Autodesk Fusion 360 part; units mm, degrees
(part 2 of 9)
  line L444 (-11.7276, 122.2942) -> (-7.3975, 119.7942)
  line L445 (-7.3975, 119.7942) -> (-3.0673, 122.2942)
  line L446 (-3.0673, 122.2942) -> (-3.0673, 127.2942)
  line L447 (-3.0673, 127.2942) -> (-7.3975, 129.7942)
  line L448 (-103.9199, 138.5933) -> (-108.25, 136.0933)
  line L449 (-108.25, 136.0933) -> (-108.25, 131.0933)
  line L450 (-108.25, 131.0933) -> (-103.9199, 128.5933)
  line L451 (-103.9199, 128.5933) -> (-99.5897, 131.0933)
  line L452 (-99.5897, 131.0933) -> (-99.5897, 136.0933)
  line L453 (-99.5897, 136.0933) -> (-103.9199, 138.5933)
  line L454 (-93.7596, 138.5933) -> (-98.0897, 136.0933)
  line L455 (-98.0897, 136.0933) -> (-98.0897, 131.0933)
  line L456 (-98.0897, 131.0933) -> (-93.7596, 128.5933)
  line L457 (-93.7596, 128.5933) -> (-89.4295, 131.0933)
  line L458 (-89.4295, 131.0933) -> (-89.4295, 136.0933)
  line L459 (-89.4295, 136.0933) -> (-93.7596, 138.5933)
  line L460 (-83.5994, 138.5933) -> (-87.9295, 136.0933)
  line L461 (-87.9295, 136.0933) -> (-87.9295, 131.0933)
  line L462 (-87.9295, 131.0933) -> (-83.5994, 128.5933)
  line L463 (-83.5994, 128.5933) -> (-79.2692, 131.0933)
  line L464 (-79.2692, 131.0933) -> (-79.2692, 136.0933)
  line L465 (-79.2692, 136.0933) -> (-83.5994, 138.5933)
  line L466 (-73.4391, 138.5933) -> (-77.7692, 136.0933)
  line L467 (-77.7692, 136.0933) -> (-77.7692, 131.0933)
  line L468 (-77.7692, 131.0933) -> (-73.4391, 128.5933)
  line L469 (-73.4391, 128.5933) -> (-69.109, 131.0933)
  line L470 (-69.109, 131.0933) -> (-69.109, 136.0933)
  line L471 (-69.109, 136.0933) -> (-73.4391, 138.5933)
  line L472 (-63.2789, 138.5933) -> (-67.609, 136.0933)
  line L473 (-67.609, 136.0933) -> (-67.609, 131.0933)
  line L474 (-67.609, 131.0933) -> (-63.2789, 128.5933)
  line L475 (-63.2789, 128.5933) -> (-58.9487, 131.0933)
  line L476 (-58.9487, 131.0933) -> (-58.9487, 136.0933)
  line L477 (-58.9487, 136.0933) -> (-63.2789, 138.5933)
  line L478 (-53.1186, 138.5933) -> (-57.4487, 136.0933)
  line L479 (-57.4487, 136.0933) -> (-57.4487, 131.0933)
  line L480 (-57.4487, 131.0933) -> (-53.1186, 128.5933)
  line L481 (-53.1186, 128.5933) -> (-48.7885, 131.0933)
  line L482 (-48.7885, 131.0933) -> (-48.7885, 136.0933)
  line L483 (-48.7885, 136.0933) -> (-53.1186, 138.5933)
  line L484 (-42.9584, 138.5933) -> (-47.2885, 136.0933)
  line L485 (-47.2885, 136.0933) -> (-47.2885, 131.0933)
  line L486 (-47.2885, 131.0933) -> (-42.9584, 128.5933)
  line L487 (-42.9584, 128.5933) -> (-38.6282, 131.0933)
  line L488 (-38.6282, 131.0933) -> (-38.6282, 136.0933)
  line L489 (-38.6282, 136.0933) -> (-42.9584, 138.5933)
  line L490 (-32.7981, 138.5933) -> (-37.1282, 136.0933)
  line L491 (-37.1282, 136.0933) -> (-37.1282, 131.0933)
  line L492 (-37.1282, 131.0933) -> (-32.7981, 128.5933)
  line L493 (-32.7981, 128.5933) -> (-28.468, 131.0933)
  line L494 (-28.468, 131.0933) -> (-28.468, 136.0933)
  line L495 (-28.468, 136.0933) -> (-32.7981, 138.5933)
  line L496 (-22.6378, 138.5933) -> (-26.968, 136.0933)
  line L497 (-26.968, 136.0933) -> (-26.968, 131.0933)
  line L498 (-26.968, 131.0933) -> (-22.6378, 128.5933)
  line L499 (-22.6378, 128.5933) -> (-18.3077, 131.0933)
  line L500 (-18.3077, 131.0933) -> (-18.3077, 136.0933)
  line L501 (-18.3077, 136.0933) -> (-22.6378, 138.5933)
  line L502 (-12.4776, 138.5933) -> (-16.8077, 136.0933)
  line L503 (-16.8077, 136.0933) -> (-16.8077, 131.0933)
  line L504 (-16.8077, 131.0933) -> (-12.4776, 128.5933)
  line L505 (-12.4776, 128.5933) -> (-8.1475, 131.0933)
  line L506 (-8.1475, 131.0933) -> (-8.1475, 136.0933)
  line L507 (-8.1475, 136.0933) -> (-12.4776, 138.5933)
  line L508 (-109, 147.3923) -> (-113.3301, 144.8923)
  line L509 (-113.3301, 144.8923) -> (-113.3301, 139.8923)
  line L510 (-113.3301, 139.8923) -> (-109, 137.3923)
  line L511 (-109, 137.3923) -> (-104.6699, 139.8923)
  line L512 (-104.6699, 139.8923) -> (-104.6699, 144.8923)
  line L513 (-104.6699, 144.8923) -> (-109, 147.3923)
  line L514 (-98.8397, 147.3923) -> (-103.1699, 144.8923)
  line L515 (-103.1699, 144.8923) -> (-103.1699, 139.8923)
  line L516 (-103.1699, 139.8923) -> (-98.8397, 137.3923)
  line L517 (-98.8397, 137.3923) -> (-94.5096, 139.8923)
  line L518 (-94.5096, 139.8923) -> (-94.5096, 144.8923)
  line L519 (-94.5096, 144.8923) -> (-98.8397, 147.3923)
  line L520 (-88.6795, 147.3923) -> (-93.0096, 144.8923)
  line L521 (-93.0096, 144.8923) -> (-93.0096, 139.8923)
  line L522 (-93.0096, 139.8923) -> (-88.6795, 137.3923)
  line L523 (-88.6795, 137.3923) -> (-84.3494, 139.8923)
  line L524 (-84.3494, 139.8923) -> (-84.3494, 144.8923)
  line L525 (-84.3494, 144.8923) -> (-88.6795, 147.3923)
  line L526 (-78.5192, 147.3923) -> (-82.8494, 144.8923)
  line L527 (-82.8494, 144.8923) -> (-82.8494, 139.8923)
  line L528 (-82.8494, 139.8923) -> (-78.5192, 137.3923)
  line L529 (-78.5192, 137.3923) -> (-74.1891, 139.8923)
  line L530 (-74.1891, 139.8923) -> (-74.1891, 144.8923)
  line L531 (-74.1891, 144.8923) -> (-78.5192, 147.3923)
  line L532 (-68.359, 147.3923) -> (-72.6891, 144.8923)
  line L533 (-72.6891, 144.8923) -> (-72.6891, 139.8923)
  line L534 (-72.6891, 139.8923) -> (-68.359, 137.3923)
  line L535 (-68.359, 137.3923) -> (-64.0289, 139.8923)
  line L536 (-64.0289, 139.8923) -> (-64.0289, 144.8923)
  line L537 (-64.0289, 144.8923) -> (-68.359, 147.3923)
  line L538 (-58.1987, 147.3923) -> (-62.5289, 144.8923)
  line L539 (-62.5289, 144.8923) -> (-62.5289, 139.8923)
  line L540 (-62.5289, 139.8923) -> (-58.1987, 137.3923)
  line L541 (-58.1987, 137.3923) -> (-53.8686, 139.8923)
  line L542 (-53.8686, 139.8923) -> (-53.8686, 144.8923)
  line L543 (-53.8686, 144.8923) -> (-58.1987, 147.3923)
  line L544 (-48.0385, 147.3923) -> (-52.3686, 144.8923)
  line L545 (-52.3686, 144.8923) -> (-52.3686, 139.8923)
  line L546 (-52.3686, 139.8923) -> (-48.0385, 137.3923)
  line L547 (-48.0385, 137.3923) -> (-43.7084, 139.8923)
  line L548 (-43.7084, 139.8923) -> (-43.7084, 144.8923)
  line L549 (-43.7084, 144.8923) -> (-48.0385, 147.3923)
  line L550 (-37.8782, 147.3923) -> (-42.2084, 144.8923)
  line L551 (-42.2084, 144.8923) -> (-42.2084, 139.8923)
  line L552 (-42.2084, 139.8923) -> (-37.8782, 137.3923)
  line L553 (-37.8782, 137.3923) -> (-33.5481, 139.8923)
  line L554 (-33.5481, 139.8923) -> (-33.5481, 144.8923)
  line L555 (-33.5481, 144.8923) -> (-37.8782, 147.3923)
  line L556 (-27.718, 147.3923) -> (-32.0481, 144.8923)
  line L557 (-32.0481, 144.8923) -> (-32.0481, 139.8923)
  line L558 (-32.0481, 139.8923) -> (-27.718, 137.3923)
  line L559 (-27.718, 137.3923) -> (-23.3878, 139.8923)
  line L560 (-23.3878, 139.8923) -> (-23.3878, 144.8923)
  line L561 (-23.3878, 144.8923) -> (-27.718, 147.3923)
  line L562 (-17.5577, 147.3923) -> (-21.8878, 144.8923)
  line L563 (-21.8878, 144.8923) -> (-21.8878, 139.8923)
  line L564 (-21.8878, 139.8923) -> (-17.5577, 137.3923)
  line L565 (-17.5577, 137.3923) -> (-13.2276, 139.8923)
  line L566 (-13.2276, 139.8923) -> (-13.2276, 144.8923)
  line L567 (-13.2276, 144.8923) -> (-17.5577, 147.3923)
  line L568 (-7.3975, 147.3923) -> (-11.7276, 144.8923)
  line L569 (-11.7276, 144.8923) -> (-11.7276, 139.8923)
  line L570 (-11.7276, 139.8923) -> (-7.3975, 137.3923)
  line L571 (-7.3975, 137.3923) -> (-3.0673, 139.8923)
  line L572 (-3.0673, 139.8923) -> (-3.0673, 144.8923)
  line L573 (-3.0673, 144.8923) -> (-7.3975, 147.3923)
  line L574 (-103.9199, 156.1913) -> (-108.25, 153.6913)
  line L575 (-108.25, 153.6913) -> (-108.25, 148.6913)
  line L576 (-108.25, 148.6913) -> (-103.9199, 146.1913)
  line L577 (-103.9199, 146.1913) -> (-99.5897, 148.6913)
  line L578 (-99.5897, 148.6913) -> (-99.5897, 153.6913)
  line L579 (-99.5897, 153.6913) -> (-103.9199, 156.1913)
  line L580 (-93.7596, 156.1913) -> (-98.0897, 153.6913)
  line L581 (-98.0897, 153.6913) -> (-98.0897, 148.6913)
  line L582 (-98.0897, 148.6913) -> (-93.7596, 146.1913)
  line L583 (-93.7596, 146.1913) -> (-89.4295, 148.6913)
  line L584 (-89.4295, 148.6913) -> (-89.4295, 153.6913)
  line L585 (-89.4295, 153.6913) -> (-93.7596, 156.1913)
  line L586 (-83.5994, 156.1913) -> (-87.9295, 153.6913)
  line L587 (-87.9295, 153.6913) -> (-87.9295, 148.6913)
  line L588 (-87.9295, 148.6913) -> (-83.5994, 146.1913)
  line L589 (-83.5994, 146.1913) -> (-79.2692, 148.6913)
  line L590 (-79.2692, 148.6913) -> (-79.2692, 153.6913)
  line L591 (-79.2692, 153.6913) -> (-83.5994, 156.1913)
  line L592 (-73.4391, 156.1913) -> (-77.7692, 153.6913)
  line L593 (-77.7692, 153.6913) -> (-77.7692, 148.6913)
  line L594 (-77.7692, 148.6913) -> (-73.4391, 146.1913)
  line L595 (-73.4391, 146.1913) -> (-69.109, 148.6913)
  line L596 (-69.109, 148.6913) -> (-69.109, 153.6913)
  line L597 (-69.109, 153.6913) -> (-73.4391, 156.1913)
  line L598 (-63.2789, 156.1913) -> (-67.609, 153.6913)
  line L599 (-67.609, 153.6913) -> (-67.609, 148.6913)
  line L600 (-67.609, 148.6913) -> (-63.2789, 146.1913)
  line L601 (-63.2789, 146.1913) -> (-58.9487, 148.6913)
  line L602 (-58.9487, 148.6913) -> (-58.9487, 153.6913)
  line L603 (-58.9487, 153.6913) -> (-63.2789, 156.1913)
  line L604 (-53.1186, 156.1913) -> (-57.4487, 153.6913)
  line L605 (-57.4487, 153.6913) -> (-57.4487, 148.6913)
  line L606 (-57.4487, 148.6913) -> (-53.1186, 146.1913)
  line L607 (-53.1186, 146.1913) -> (-48.7885, 148.6913)
  line L608 (-48.7885, 148.6913) -> (-48.7885, 153.6913)
  line L609 (-48.7885, 153.6913) -> (-53.1186, 156.1913)
  line L610 (-42.9584, 156.1913) -> (-47.2885, 153.6913)
  line L611 (-47.2885, 153.6913) -> (-47.2885, 148.6913)
  line L612 (-47.2885, 148.6913) -> (-42.9584, 146.1913)
  line L613 (-42.9584, 146.1913) -> (-38.6282, 148.6913)
  line L614 (-38.6282, 148.6913) -> (-38.6282, 153.6913)
  line L615 (-38.6282, 153.6913) -> (-42.9584, 156.1913)
  line L616 (-32.7981, 156.1913) -> (-37.1282, 153.6913)
  line L617 (-37.1282, 153.6913) -> (-37.1282, 148.6913)
  line L618 (-37.1282, 148.6913) -> (-32.7981, 146.1913)
  line L619 (-32.7981, 146.1913) -> (-28.468, 148.6913)
  line L620 (-28.468, 148.6913) -> (-28.468, 153.6913)
  line L621 (-28.468, 153.6913) -> (-32.7981, 156.1913)
  line L622 (-22.6378, 156.1913) -> (-26.968, 153.6913)
  line L623 (-26.968, 153.6913) -> (-26.968, 148.6913)
  line L624 (-26.968, 148.6913) -> (-22.6378, 146.1913)
  line L625 (-22.6378, 146.1913) -> (-18.3077, 148.6913)
  line L626 (-18.3077, 148.6913) -> (-18.3077, 153.6913)
  line L627 (-18.3077, 153.6913) -> (-22.6378, 156.1913)
  line L628 (-12.4776, 156.1913) -> (-16.8077, 153.6913)
  line L629 (-16.8077, 153.6913) -> (-16.8077, 148.6913)
  line L630 (-16.8077, 148.6913) -> (-12.4776, 146.1913)
  line L631 (-12.4776, 146.1913) -> (-8.1475, 148.6913)
  line L632 (-8.1475, 148.6913) -> (-8.1475, 153.6913)
  line L633 (-8.1475, 153.6913) -> (-12.4776, 156.1913)
extrude "拉伸21" cut sketch "草图20" against normal blind 3 contours L4 L5 L6 L7 L8 L9 | L10 L11 L12 L13 L14 L15 | L16 L17 L18 L19 L20 L21 | L22 L23 L24 L25 L26 L27 | L28 L29 L30 L31 L32 L33 | L34 L35 L36 L37 L38 L39 | L40 L41 L42 L43 L44 L45 | L46 L47 L48 L49 L50 L51 | L52 L53 L54 L55 L56 L57 | L58 L59 L60 L61 L62 L63 | L64 L65 L66 L67 L68 L69 | L70 L71 L72 L73 L74 L75 | L76 L77 L78 L79 L80 L81 | L82 L83 L84 L85 L86 L87 | L88 L89 L90 L91 L92 L93 | L94 L95 L96 L97 L98 L99 | L100 L101 L102 L103 L104 L105 | L106 L107 L108 L109 L110 L111 | L112 L113 L114 L115 L116 L117 | L118 L119 L120 L121 L122 L123 | L124 L125 L126 L127 L128 L129 | L130 L131 L132 L133 L134 L135 | L136 L137 L138 L139 L140 L141 | L142 L143 L144 L145 L146 L147 | L148 L149 L150 L151 L152 L153 | L154 L155 L156 L157 L158 L159 | L160 L161 L162 L163 L164 L165 | L166 L167 L168 L169 L170 L171 | L172 L173 L174 L175 L176 L177 | L178 L179 L180 L181 L182 L183 | L184 L185 L186 L187 L188 L189 | L190 L191 L192 L193 L194 L195 | L196 L197 L198 L199 L200 L201 | L202 L203 L204 L205 L206 L207 | L208 L209 L210 L211 L212 L213 | L214 L215 L216 L217 L218 L219 | L220 L221 L222 L223 L224 L225 | L226 L227 L228 L229 L230 L231 | L232 L233 L234 L235 L236 L237 | L238 L239 L240 L241 L242 L243 | L244 L245 L246 L247 L248 L249 | L250 L251 L252 L253 L254 L255 | L256 L257 L258 L259 L260 L261 | L262 L263 L264 L265 L266 L267 | L268 L269 L270 L271 L272 L273 | L274 L275 L276 L277 L278 L279 | L280 L281 L282 L283 L284 L285 | L286 L287 L288 L289 L290 L291 | L292 L293 L294 L295 L296 L297 | L298 L299 L300 L301 L302 L303 | L304 L305 L306 L307 L308 L309 | L310 L311 L312 L313 L314 L315 | L316 L317 L318 L319 L320 L321 | L322 L323 L324 L325 L326 L327 | L328 L329 L330 L331 L332 L333 | L334 L335 L336 L337 L338 L339 | L340 L341 L342 L343 L344 L345 | L346 L347 L348 L349 L350 L351 | L352 L353 L354 L355 L356 L357 | L358 L359 L360 L361 L362 L363 | L364 L365 L366 L367 L368 L369 | L370 L371 L372 L373 L374 L375 | L376 L377 L378 L379 L380 L381 | L382 L383 L384 L385 L386 L387 | L388 L389 L390 L391 L392 L393 | L394 L395 L396 L397 L398 L399 | L400 L401 L402 L403 L404 L405 | L406 L407 L408 L409 L410 L411 | L412 L413 L414 L415 L416 L417 | L418 L419 L420 L421 L422 L423 | L424 L425 L426 L427 L428 L429 | L430 L431 L432 L433 L434 L435 | L436 L437 L438 L439 L440 L441 | L442 L443 L444 L445 L446 L447 | L448 L449 L450 L451 L452 L453 | L454 L455 L456 L457 L458 L459 | L460 L461 L462 L463 L464 L465 | L466 L467 L468 L469 L470 L471 | L472 L473 L474 L475 L476 L477 | L478 L479 L480 L481 L482 L483 | L484 L485 L486 L487 L488 L489 | L490 L491 L492 L493 L494 L495 | L496 L497 L498 L499 L500 L501 | L502 L503 L504 L505 L506 L507 | L508 L509 L510 L511 L512 L513 | L514 L515 L516 L517 L518 L519 | L520 L521 L522 L523 L524 L525 | L526 L527 L528 L529 L530 L531 | L532 L533 L534 L535 L536 L537 | L538 L539 L540 L541 L542 L543 | L544 L545 L546 L547 L548 L549 | L550 L551 L552 L553 L554 L555 | L556 L557 L558 L559 L560 L561 | L562 L563 L564 L565 L566 L567 | L568 L569 L570 L571 L572 L573 | L574 L575 L576 L577 L578 L579 | L580 L581 L582 L583 L584 L585 | L586 L587 L588 L589 L590 L591 | L592 L593 L594 L595 L596 L597 | L598 L599 L600 L601 L602 L603 | L604 L605 L606 L607 L608 L609 | L610 L611 L612 L613 L614 L615 | L616 L617 L618 L619 L620 L621 | L622 L623 L624 L625 L626 L627 | L628 L629 L630 L631 L632 L633 bodies 1
sketch "草图21" plane through (0, 116, 0) normal (0, -1, 0) x (1, 0, 0)
  line L0 (3.9913, 65) -> (4, 65)
  line L1 (4, 65) -> (4, 160)
  line L2 (4, 160) -> (-116, 160)
  line L3 (-116, 160) -> (-116, 0)
  line L4 (-116, 0) -> (3.9913, 0)
  line L5 (3.9913, 0) -> (3.9913, 65)
  line L6 (-103.9199, 20.799) -> (-108.25, 18.299)
  line L7 (-108.25, 18.299) -> (-108.25, 13.299)
  line L8 (-108.25, 13.299) -> (-103.9199, 10.799)
  line L9 (-103.9199, 10.799) -> (-99.5897, 13.299)
  line L10 (-99.5897, 13.299) -> (-99.5897, 18.299)
  line L11 (-99.5897, 18.299) -> (-103.9199, 20.799)
  line L12 (-93.7596, 20.799) -> (-98.0897, 18.299)
  line L13 (-98.0897, 18.299) -> (-98.0897, 13.299)
  line L14 (-98.0897, 13.299) -> (-93.7596, 10.799)
  line L15 (-93.7596, 10.799) -> (-89.4295, 13.299)
  line L16 (-89.4295, 13.299) -> (-89.4295, 18.299)
  line L17 (-89.4295, 18.299) -> (-93.7596, 20.799)
  line L18 (-83.5994, 20.799) -> (-87.9295, 18.299)
  line L19 (-87.9295, 18.299) -> (-87.9295, 13.299)
  line L20 (-87.9295, 13.299) -> (-83.5994, 10.799)
  line L21 (-83.5994, 10.799) -> (-79.2692, 13.299)
  line L22 (-79.2692, 13.299) -> (-79.2692, 18.299)
  line L23 (-79.2692, 18.299) -> (-83.5994, 20.799)
  line L24 (-73.4391, 20.799) -> (-77.7692, 18.299)
  line L25 (-77.7692, 18.299) -> (-77.7692, 13.299)
  line L26 (-77.7692, 13.299) -> (-73.4391, 10.799)
  line L27 (-73.4391, 10.799) -> (-69.109, 13.299)
  line L28 (-69.109, 13.299) -> (-69.109, 18.299)
  line L29 (-69.109, 18.299) -> (-73.4391, 20.799)
  line L30 (-63.2789, 20.799) -> (-67.609, 18.299)
  line L31 (-67.609, 18.299) -> (-67.609, 13.299)
  line L32 (-67.609, 13.299) -> (-63.2789, 10.799)
  line L33 (-63.2789, 10.799) -> (-58.9487, 13.299)
  line L34 (-58.9487, 13.299) -> (-58.9487, 18.299)
  line L35 (-58.9487, 18.299) -> (-63.2789, 20.799)
  line L36 (-53.1186, 20.799) -> (-57.4487, 18.299)
  line L37 (-57.4487, 18.299) -> (-57.4487, 13.299)
  line L38 (-57.4487, 13.299) -> (-53.1186, 10.799)
  line L39 (-53.1186, 10.799) -> (-48.7885, 13.299)
  line L40 (-48.7885, 13.299) -> (-48.7885, 18.299)
  line L41 (-48.7885, 18.299) -> (-53.1186, 20.799)
  line L42 (-42.9584, 20.799) -> (-47.2885, 18.299)
  line L43 (-47.2885, 18.299) -> (-47.2885, 13.299)
  line L44 (-47.2885, 13.299) -> (-42.9584, 10.799)
  line L45 (-42.9584, 10.799) -> (-38.6282, 13.299)
  line L46 (-38.6282, 13.299) -> (-38.6282, 18.299)
  line L47 (-38.6282, 18.299) -> (-42.9584, 20.799)
  line L48 (-32.7981, 20.799) -> (-37.1282, 18.299)
  line L49 (-37.1282, 18.299) -> (-37.1282, 13.299)
  line L50 (-37.1282, 13.299) -> (-32.7981, 10.799)
  line L51 (-32.7981, 10.799) -> (-28.468, 13.299)
  line L52 (-28.468, 13.299) -> (-28.468, 18.299)
  line L53 (-28.468, 18.299) -> (-32.7981, 20.799)
  line L54 (-22.6378, 20.799) -> (-26.968, 18.299)
  line L55 (-26.968, 18.299) -> (-26.968, 13.299)
  line L56 (-26.968, 13.299) -> (-22.6378, 10.799)
  line L57 (-22.6378, 10.799) -> (-18.3077, 13.299)
  line L58 (-18.3077, 13.299) -> (-18.3077, 18.299)
  line L59 (-18.3077, 18.299) -> (-22.6378, 20.799)
  line L60 (-12.4776, 20.799) -> (-16.8077, 18.299)
  line L61 (-16.8077, 18.299) -> (-16.8077, 13.299)
  line L62 (-16.8077, 13.299) -> (-12.4776, 10.799)
  line L63 (-12.4776, 10.799) -> (-8.1475, 13.299)
  line L64 (-8.1475, 13.299) -> (-8.1475, 18.299)
  line L65 (-8.1475, 18.299) -> (-12.4776, 20.799)
  line L66 (-109, 29.5981) -> (-113.3301, 27.0981)
  line L67 (-113.3301, 27.0981) -> (-113.3301, 22.0981)
  line L68 (-113.3301, 22.0981) -> (-109, 19.5981)
  line L69 (-109, 19.5981) -> (-104.6699, 22.0981)
  line L70 (-104.6699, 22.0981) -> (-104.6699, 27.0981)
  line L71 (-104.6699, 27.0981) -> (-109, 29.5981)
  line L72 (-98.8397, 29.5981) -> (-103.1699, 27.0981)
  line L73 (-103.1699, 27.0981) -> (-103.1699, 22.0981)
  line L74 (-103.1699, 22.0981) -> (-98.8397, 19.5981)
  line L75 (-98.8397, 19.5981) -> (-94.5096, 22.0981)
  line L76 (-94.5096, 22.0981) -> (-94.5096, 27.0981)
  line L77 (-94.5096, 27.0981) -> (-98.8397, 29.5981)
  line L78 (-88.6795, 29.5981) -> (-93.0096, 27.0981)
  line L79 (-93.0096, 27.0981) -> (-93.0096, 22.0981)
  line L80 (-93.0096, 22.0981) -> (-88.6795, 19.5981)
  line L81 (-88.6795, 19.5981) -> (-84.3494, 22.0981)
  line L82 (-84.3494, 22.0981) -> (-84.3494, 27.0981)
  line L83 (-84.3494, 27.0981) -> (-88.6795, 29.5981)
  line L84 (-78.5192, 29.5981) -> (-82.8494, 27.0981)
  line L85 (-82.8494, 27.0981) -> (-82.8494, 22.0981)
  line L86 (-82.8494, 22.0981) -> (-78.5192, 19.5981)
  line L87 (-78.5192, 19.5981) -> (-74.1891, 22.0981)
  line L88 (-74.1891, 22.0981) -> (-74.1891, 27.0981)
  line L89 (-74.1891, 27.0981) -> (-78.5192, 29.5981)
  line L90 (-68.359, 29.5981) -> (-72.6891, 27.0981)
  line L91 (-72.6891, 27.0981) -> (-72.6891, 22.0981)
  line L92 (-72.6891, 22.0981) -> (-68.359, 19.5981)
  line L93 (-68.359, 19.5981) -> (-64.0289, 22.0981)
  line L94 (-64.0289, 22.0981) -> (-64.0289, 27.0981)
  line L95 (-64.0289, 27.0981) -> (-68.359, 29.5981)
  line L96 (-58.1987, 29.5981) -> (-62.5289, 27.0981)
  line L97 (-62.5289, 27.0981) -> (-62.5289, 22.0981)
  line L98 (-62.5289, 22.0981) -> (-58.1987, 19.5981)
  line L99 (-58.1987, 19.5981) -> (-53.8686, 22.0981)
  line L100 (-53.8686, 22.0981) -> (-53.8686, 27.0981)
  line L101 (-53.8686, 27.0981) -> (-58.1987, 29.5981)
  line L102 (-48.0385, 29.5981) -> (-52.3686, 27.0981)
  line L103 (-52.3686, 27.0981) -> (-52.3686, 22.0981)
  line L104 (-52.3686, 22.0981) -> (-48.0385, 19.5981)
  line L105 (-48.0385, 19.5981) -> (-43.7084, 22.0981)
  line L106 (-43.7084, 22.0981) -> (-43.7084, 27.0981)
  line L107 (-43.7084, 27.0981) -> (-48.0385, 29.5981)
  line L108 (-37.8782, 29.5981) -> (-42.2084, 27.0981)
  line L109 (-42.2084, 27.0981) -> (-42.2084, 22.0981)
  line L110 (-42.2084, 22.0981) -> (-37.8782, 19.5981)
  line L111 (-37.8782, 19.5981) -> (-33.5481, 22.0981)
  line L112 (-33.5481, 22.0981) -> (-33.5481, 27.0981)
  line L113 (-33.5481, 27.0981) -> (-37.8782, 29.5981)
  line L114 (-27.718, 29.5981) -> (-32.0481, 27.0981)
  line L115 (-32.0481, 27.0981) -> (-32.0481, 22.0981)
  line L116 (-32.0481, 22.0981) -> (-27.718, 19.5981)
  line L117 (-27.718, 19.5981) -> (-23.3878, 22.0981)
  line L118 (-23.3878, 22.0981) -> (-23.3878, 27.0981)
  line L119 (-23.3878, 27.0981) -> (-27.718, 29.5981)
  line L120 (-17.5577, 29.5981) -> (-21.8878, 27.0981)
  line L121 (-21.8878, 27.0981) -> (-21.8878, 22.0981)
  line L122 (-21.8878, 22.0981) -> (-17.5577, 19.5981)
  line L123 (-17.5577, 19.5981) -> (-13.2276, 22.0981)
  line L124 (-13.2276, 22.0981) -> (-13.2276, 27.0981)
  line L125 (-13.2276, 27.0981) -> (-17.5577, 29.5981)
  line L126 (-7.3975, 29.5981) -> (-11.7276, 27.0981)
  line L127 (-11.7276, 27.0981) -> (-11.7276, 22.0981)
  line L128 (-11.7276, 22.0981) -> (-7.3975, 19.5981)
  line L129 (-7.3975, 19.5981) -> (-3.0673, 22.0981)
  line L130 (-3.0673, 22.0981) -> (-3.0673, 27.0981)
  line L131 (-3.0673, 27.0981) -> (-7.3975, 29.5981)
  line L132 (-103.9199, 38.3971) -> (-108.25, 35.8971)
  line L133 (-108.25, 35.8971) -> (-108.25, 30.8971)
  line L134 (-108.25, 30.8971) -> (-103.9199, 28.3971)
  line L135 (-103.9199, 28.3971) -> (-99.5897, 30.8971)
  line L136 (-99.5897, 30.8971) -> (-99.5897, 35.8971)
  line L137 (-99.5897, 35.8971) -> (-103.9199, 38.3971)
  line L138 (-93.7596, 38.3971) -> (-98.0897, 35.8971)
  line L139 (-98.0897, 35.8971) -> (-98.0897, 30.8971)
  line L140 (-98.0897, 30.8971) -> (-93.7596, 28.3971)
  line L141 (-93.7596, 28.3971) -> (-89.4295, 30.8971)
  line L142 (-89.4295, 30.8971) -> (-89.4295, 35.8971)
  line L143 (-89.4295, 35.8971) -> (-93.7596, 38.3971)
  line L144 (-83.5994, 38.3971) -> (-87.9295, 35.8971)
  line L145 (-87.9295, 35.8971) -> (-87.9295, 30.8971)
  line L146 (-87.9295, 30.8971) -> (-83.5994, 28.3971)
  line L147 (-83.5994, 28.3971) -> (-79.2692, 30.8971)
  line L148 (-79.2692, 30.8971) -> (-79.2692, 35.8971)
  line L149 (-79.2692, 35.8971) -> (-83.5994, 38.3971)
  line L150 (-73.4391, 38.3971) -> (-77.7692, 35.8971)
  line L151 (-77.7692, 35.8971) -> (-77.7692, 30.8971)
  line L152 (-77.7692, 30.8971) -> (-73.4391, 28.3971)
  line L153 (-73.4391, 28.3971) -> (-69.109, 30.8971)
  line L154 (-69.109, 30.8971) -> (-69.109, 35.8971)
  line L155 (-69.109, 35.8971) -> (-73.4391, 38.3971)
  line L156 (-63.2789, 38.3971) -> (-67.609, 35.8971)
  line L157 (-67.609, 35.8971) -> (-67.609, 30.8971)
  line L158 (-67.609, 30.8971) -> (-63.2789, 28.3971)
  line L159 (-63.2789, 28.3971) -> (-58.9487, 30.8971)
  line L160 (-58.9487, 30.8971) -> (-58.9487, 35.8971)
  line L161 (-58.9487, 35.8971) -> (-63.2789, 38.3971)
  line L162 (-53.1186, 38.3971) -> (-57.4487, 35.8971)
  line L163 (-57.4487, 35.8971) -> (-57.4487, 30.8971)
  line L164 (-57.4487, 30.8971) -> (-53.1186, 28.3971)
  line L165 (-53.1186, 28.3971) -> (-48.7885, 30.8971)
  line L166 (-48.7885, 30.8971) -> (-48.7885, 35.8971)
  line L167 (-48.7885, 35.8971) -> (-53.1186, 38.3971)
  line L168 (-42.9584, 38.3971) -> (-47.2885, 35.8971)
  line L169 (-47.2885, 35.8971) -> (-47.2885, 30.8971)
  line L170 (-47.2885, 30.8971) -> (-42.9584, 28.3971)
  line L171 (-42.9584, 28.3971) -> (-38.6282, 30.8971)
  line L172 (-38.6282, 30.8971) -> (-38.6282, 35.8971)
  line L173 (-38.6282, 35.8971) -> (-42.9584, 38.3971)
  line L174 (-32.7981, 38.3971) -> (-37.1282, 35.8971)
  line L175 (-37.1282, 35.8971) -> (-37.1282, 30.8971)
  line L176 (-37.1282, 30.8971) -> (-32.7981, 28.3971)
  line L177 (-32.7981, 28.3971) -> (-28.468, 30.8971)
  line L178 (-28.468, 30.8971) -> (-28.468, 35.8971)
  line L179 (-28.468, 35.8971) -> (-32.7981, 38.3971)
  line L180 (-22.6378, 38.3971) -> (-26.968, 35.8971)
  line L181 (-26.968, 35.8971) -> (-26.968, 30.8971)
  line L182 (-26.968, 30.8971) -> (-22.6378, 28.3971)
  line L183 (-22.6378, 28.3971) -> (-18.3077, 30.8971)
  line L184 (-18.3077, 30.8971) -> (-18.3077, 35.8971)
  line L185 (-18.3077, 35.8971) -> (-22.6378, 38.3971)
  line L186 (-12.4776, 38.3971) -> (-16.8077, 35.8971)
  line L187 (-16.8077, 35.8971) -> (-16.8077, 30.8971)
  line L188 (-16.8077, 30.8971) -> (-12.4776, 28.3971)
  line L189 (-12.4776, 28.3971) -> (-8.1475, 30.8971)
  line L190 (-8.1475, 30.8971) -> (-8.1475, 35.8971)
  line L191 (-8.1475, 35.8971) -> (-12.4776, 38.3971)
  line L192 (-109, 47.1962) -> (-113.3301, 44.6962)
  line L193 (-113.3301, 44.6962) -> (-113.3301, 39.6962)
  line L194 (-113.3301, 39.6962) -> (-109, 37.1962)
  line L195 (-109, 37.1962) -> (-104.6699, 39.6962)
  line L196 (-104.6699, 39.6962) -> (-104.6699, 44.6962)
  line L197 (-104.6699, 44.6962) -> (-109, 47.1962)
  line L198 (-98.8397, 47.1962) -> (-103.1699, 44.6962)
  line L199 (-103.1699, 44.6962) -> (-103.1699, 39.6962)
  line L200 (-103.1699, 39.6962) -> (-98.8397, 37.1962)
  line L201 (-98.8397, 37.1962) -> (-94.5096, 39.6962)
  line L202 (-94.5096, 39.6962) -> (-94.5096, 44.6962)
  line L203 (-94.5096, 44.6962) -> (-98.8397, 47.1962)
  line L204 (-88.6795, 47.1962) -> (-93.0096, 44.6962)
  line L205 (-93.0096, 44.6962) -> (-93.0096, 39.6962)
  line L206 (-93.0096, 39.6962) -> (-88.6795, 37.1962)
  line L207 (-88.6795, 37.1962) -> (-84.3494, 39.6962)
  line L208 (-84.3494, 39.6962) -> (-84.3494, 44.6962)
  line L209 (-84.3494, 44.6962) -> (-88.6795, 47.1962)
  line L210 (-78.5192, 47.1962) -> (-82.8494, 44.6962)
  line L211 (-82.8494, 44.6962) -> (-82.8494, 39.6962)
  line L212 (-82.8494, 39.6962) -> (-78.5192, 37.1962)
  line L213 (-78.5192, 37.1962) -> (-74.1891, 39.6962)
  line L214 (-74.1891, 39.6962) -> (-74.1891, 44.6962)
  line L215 (-74.1891, 44.6962) -> (-78.5192, 47.1962)
  line L216 (-68.359, 47.1962) -> (-72.6891, 44.6962)
  line L217 (-72.6891, 44.6962) -> (-72.6891, 39.6962)
  line L218 (-72.6891, 39.6962) -> (-68.359, 37.1962)
  line L219 (-68.359, 37.1962) -> (-64.0289, 39.6962)
  line L220 (-64.0289, 39.6962) -> (-64.0289, 44.6962)
  line L221 (-64.0289, 44.6962) -> (-68.359, 47.1962)
  line L222 (-58.1987, 47.1962) -> (-62.5289, 44.6962)
  line L223 (-62.5289, 44.6962) -> (-62.5289, 39.6962)
  line L224 (-62.5289, 39.6962) -> (-58.1987, 37.1962)
  line L225 (-58.1987, 37.1962) -> (-53.8686, 39.6962)
  line L226 (-53.8686, 39.6962) -> (-53.8686, 44.6962)
  line L227 (-53.8686, 44.6962) -> (-58.1987, 47.1962)
  line L228 (-48.0385, 47.1962) -> (-52.3686, 44.6962)
  line L229 (-52.3686, 44.6962) -> (-52.3686, 39.6962)
  line L230 (-52.3686, 39.6962) -> (-48.0385, 37.1962)
  line L231 (-48.0385, 37.1962) -> (-43.7084, 39.6962)
  line L232 (-43.7084, 39.6962) -> (-43.7084, 44.6962)
  line L233 (-43.7084, 44.6962) -> (-48.0385, 47.1962)
  line L234 (-37.8782, 47.1962) -> (-42.2084, 44.6962)
  line L235 (-42.2084, 44.6962) -> (-42.2084, 39.6962)
  line L236 (-42.2084, 39.6962) -> (-37.8782, 37.1962)
  line L237 (-37.8782, 37.1962) -> (-33.5481, 39.6962)
  line L238 (-33.5481, 39.6962) -> (-33.5481, 44.6962)
  line L239 (-33.5481, 44.6962) -> (-37.8782, 47.1962)
  line L240 (-27.718, 47.1962) -> (-32.0481, 44.6962)
  line L241 (-32.0481, 44.6962) -> (-32.0481, 39.6962)
  line L242 (-32.0481, 39.6962) -> (-27.718, 37.1962)
  line L243 (-27.718, 37.1962) -> (-23.3878, 39.6962)
  line L244 (-23.3878, 39.6962) -> (-23.3878, 44.6962)
  line L245 (-23.3878, 44.6962) -> (-27.718, 47.1962)
  line L246 (-17.5577, 47.1962) -> (-21.8878, 44.6962)
  line L247 (-21.8878, 44.6962) -> (-21.8878, 39.6962)
  line L248 (-21.8878, 39.6962) -> (-17.5577, 37.1962)
  line L249 (-17.5577, 37.1962) -> (-13.2276, 39.6962)
  line L250 (-13.2276, 39.6962) -> (-13.2276, 44.6962)
  line L251 (-13.2276, 44.6962) -> (-17.5577, 47.1962)
  line L252 (-7.3975, 47.1962) -> (-11.7276, 44.6962)
  line L253 (-11.7276, 44.6962) -> (-11.7276, 39.6962)
  line L254 (-11.7276, 39.6962) -> (-7.3975, 37.1962)
  line L255 (-7.3975, 37.1962) -> (-3.0673, 39.6962)
  line L256 (-3.0673, 39.6962) -> (-3.0673, 44.6962)
  line L257 (-3.0673, 44.6962) -> (-7.3975, 47.1962)
  line L258 (-103.9199, 55.9952) -> (-108.25, 53.4952)
  line L259 (-108.25, 53.4952) -> (-108.25, 48.4952)
  line L260 (-108.25, 48.4952) -> (-103.9199, 45.9952)
  line L261 (-103.9199, 45.9952) -> (-99.5897, 48.4952)
  line L262 (-99.5897, 48.4952) -> (-99.5897, 53.4952)
  line L263 (-99.5897, 53.4952) -> (-103.9199, 55.9952)
  line L264 (-93.7596, 55.9952) -> (-98.0897, 53.4952)
  line L265 (-98.0897, 53.4952) -> (-98.0897, 48.4952)
  line L266 (-98.0897, 48.4952) -> (-93.7596, 45.9952)
  line L267 (-93.7596, 45.9952) -> (-89.4295, 48.4952)
  line L268 (-89.4295, 48.4952) -> (-89.4295, 53.4952)
  line L269 (-89.4295, 53.4952) -> (-93.7596, 55.9952)
  line L270 (-83.5994, 55.9952) -> (-87.9295, 53.4952)
  line L271 (-87.9295, 53.4952) -> (-87.9295, 48.4952)
  line L272 (-87.9295, 48.4952) -> (-83.5994, 45.9952)
  line L273 (-83.5994, 45.9952) -> (-79.2692, 48.4952)
  line L274 (-79.2692, 48.4952) -> (-79.2692, 53.4952)
  line L275 (-79.2692, 53.4952) -> (-83.5994, 55.9952)
  line L276 (-73.4391, 55.9952) -> (-77.7692, 53.4952)
  line L277 (-77.7692, 53.4952) -> (-77.7692, 48.4952)
  line L278 (-77.7692, 48.4952) -> (-73.4391, 45.9952)
  line L279 (-73.4391, 45.9952) -> (-69.109, 48.4952)
  line L280 (-69.109, 48.4952) -> (-69.109, 53.4952)
  line L281 (-69.109, 53.4952) -> (-73.4391, 55.9952)
  line L282 (-63.2789, 55.9952) -> (-67.609, 53.4952)
  line L283 (-67.609, 53.4952) -> (-67.609, 48.4952)
  line L284 (-67.609, 48.4952) -> (-63.2789, 45.9952)
  line L285 (-63.2789, 45.9952) -> (-58.9487, 48.4952)
  line L286 (-58.9487, 48.4952) -> (-58.9487, 53.4952)
  line L287 (-58.9487, 53.4952) -> (-63.2789, 55.9952)
  line L288 (-53.1186, 55.9952) -> (-57.4487, 53.4952)
  line L289 (-57.4487, 53.4952) -> (-57.4487, 48.4952)
  line L290 (-57.4487, 48.4952) -> (-53.1186, 45.9952)
  line L291 (-53.1186, 45.9952) -> (-48.7885, 48.4952)
  line L292 (-48.7885, 48.4952) -> (-48.7885, 53.4952)
  line L293 (-48.7885, 53.4952) -> (-53.1186, 55.9952)
  line L294 (-42.9584, 55.9952) -> (-47.2885, 53.4952)
  line L295 (-47.2885, 53.4952) -> (-47.2885, 48.4952)
  line L296 (-47.2885, 48.4952) -> (-42.9584, 45.9952)
  line L297 (-42.9584, 45.9952) -> (-38.6282, 48.4952)
  line L298 (-38.6282, 48.4952) -> (-38.6282, 53.4952)
  line L299 (-38.6282, 53.4952) -> (-42.9584, 55.9952)
  line L300 (-32.7981, 55.9952) -> (-37.1282, 53.4952)
  line L301 (-37.1282, 53.4952) -> (-37.1282, 48.4952)
  line L302 (-37.1282, 48.4952) -> (-32.7981, 45.9952)
  line L303 (-32.7981, 45.9952) -> (-28.468, 48.4952)
  line L304 (-28.468, 48.4952) -> (-28.468, 53.4952)
  line L305 (-28.468, 53.4952) -> (-32.7981, 55.9952)
  line L306 (-22.6378, 55.9952) -> (-26.968, 53.4952)
  line L307 (-26.968, 53.4952) -> (-26.968, 48.4952)
  line L308 (-26.968, 48.4952) -> (-22.6378, 45.9952)
  line L309 (-22.6378, 45.9952) -> (-18.3077, 48.4952)
  line L310 (-18.3077, 48.4952) -> (-18.3077, 53.4952)
  line L311 (-18.3077, 53.4952) -> (-22.6378, 55.9952)
  line L312 (-12.4776, 55.9952) -> (-16.8077, 53.4952)
  line L313 (-16.8077, 53.4952) -> (-16.8077, 48.4952)
  line L314 (-16.8077, 48.4952) -> (-12.4776, 45.9952)
  line L315 (-12.4776, 45.9952) -> (-8.1475, 48.4952)
  line L316 (-8.1475, 48.4952) -> (-8.1475, 53.4952)
  line L317 (-8.1475, 53.4952) -> (-12.4776, 55.9952)
  line L318 (-109, 64.7942) -> (-113.3301, 62.2942)
  line L319 (-113.3301, 62.2942) -> (-113.3301, 57.2942)
  line L320 (-113.3301, 57.2942) -> (-109, 54.7942)
  line L321 (-109, 54.7942) -> (-104.6699, 57.2942)
  line L322 (-104.6699, 57.2942) -> (-104.6699, 62.2942)
  line L323 (-104.6699, 62.2942) -> (-109, 64.7942)
  line L324 (-98.8397, 64.7942) -> (-103.1699, 62.2942)
  line L325 (-103.1699, 62.2942) -> (-103.1699, 57.2942)
  line L326 (-103.1699, 57.2942) -> (-98.8397, 54.7942)
  line L327 (-98.8397, 54.7942) -> (-94.5096, 57.2942)
  line L328 (-94.5096, 57.2942) -> (-94.5096, 62.2942)
  line L329 (-94.5096, 62.2942) -> (-98.8397, 64.7942)
  line L330 (-88.6795, 64.7942) -> (-93.0096, 62.2942)
  line L331 (-93.0096, 62.2942) -> (-93.0096, 57.2942)
  line L332 (-93.0096, 57.2942) -> (-88.6795, 54.7942)
  line L333 (-88.6795, 54.7942) -> (-84.3494, 57.2942)
  line L334 (-84.3494, 57.2942) -> (-84.3494, 62.2942)
  line L335 (-84.3494, 62.2942) -> (-88.6795, 64.7942)
  line L336 (-78.5192, 64.7942) -> (-82.8494, 62.2942)
  line L337 (-82.8494, 62.2942) -> (-82.8494, 57.2942)
  line L338 (-82.8494, 57.2942) -> (-78.5192, 54.7942)
  line L339 (-78.5192, 54.7942) -> (-74.1891, 57.2942)
  line L340 (-74.1891, 57.2942) -> (-74.1891, 62.2942)
  line L341 (-74.1891, 62.2942) -> (-78.5192, 64.7942)
  line L342 (-68.359, 64.7942) -> (-72.6891, 62.2942)
  line L343 (-72.6891, 62.2942) -> (-72.6891, 57.2942)
  line L344 (-72.6891, 57.2942) -> (-68.359, 54.7942)
  line L345 (-68.359, 54.7942) -> (-64.0289, 57.2942)
  line L346 (-64.0289, 57.2942) -> (-64.0289, 62.2942)
  line L347 (-64.0289, 62.2942) -> (-68.359, 64.7942)
  line L348 (-58.1987, 64.7942) -> (-62.5289, 62.2942)
  line L349 (-62.5289, 62.2942) -> (-62.5289, 57.2942)
  line L350 (-62.5289, 57.2942) -> (-58.1987, 54.7942)
  line L351 (-58.1987, 54.7942) -> (-53.8686, 57.2942)
  line L352 (-53.8686, 57.2942) -> (-53.8686, 62.2942)
  line L353 (-53.8686, 62.2942) -> (-58.1987, 64.7942)
  line L354 (-48.0385, 64.7942) -> (-52.3686, 62.2942)
  line L355 (-52.3686, 62.2942) -> (-52.3686, 57.2942)
  line L356 (-52.3686, 57.2942) -> (-48.0385, 54.7942)
  line L357 (-48.0385, 54.7942) -> (-43.7084, 57.2942)
  line L358 (-43.7084, 57.2942) -> (-43.7084, 62.2942)
  line L359 (-43.7084, 62.2942) -> (-48.0385, 64.7942)
  line L360 (-37.8782, 64.7942) -> (-42.2084, 62.2942)
  line L361 (-42.2084, 62.2942) -> (-42.2084, 57.2942)
  line L362 (-42.2084, 57.2942) -> (-37.8782, 54.7942)
  line L363 (-37.8782, 54.7942) -> (-33.5481, 57.2942)
  line L364 (-33.5481, 57.2942) -> (-33.5481, 62.2942)
  line L365 (-33.5481, 62.2942) -> (-37.8782, 64.7942)
  line L366 (-27.718, 64.7942) -> (-32.0481, 62.2942)
  line L367 (-32.0481, 62.2942) -> (-32.0481, 57.2942)
  line L368 (-32.0481, 57.2942) -> (-27.718, 54.7942)
  line L369 (-27.718, 54.7942) -> (-23.3878, 57.2942)
  line L370 (-23.3878, 57.2942) -> (-23.3878, 62.2942)
  line L371 (-23.3878, 62.2942) -> (-27.718, 64.7942)
  line L372 (-17.5577, 64.7942) -> (-21.8878, 62.2942)
  line L373 (-21.8878, 62.2942) -> (-21.8878, 57.2942)
  line L374 (-21.8878, 57.2942) -> (-17.5577, 54.7942)
  line L375 (-17.5577, 54.7942) -> (-13.2276, 57.2942)
  line L376 (-13.2276, 57.2942) -> (-13.2276, 62.2942)
  line L377 (-13.2276, 62.2942) -> (-17.5577, 64.7942)
  line L378 (-7.3975, 64.7942) -> (-11.7276, 62.2942)
  line L379 (-11.7276, 62.2942) -> (-11.7276, 57.2942)
  line L380 (-11.7276, 57.2942) -> (-7.3975, 54.7942)
  line L381 (-7.3975, 54.7942) -> (-3.0673, 57.2942)
  line L382 (-3.0673, 57.2942) -> (-3.0673, 62.2942)
  line L383 (-3.0673, 62.2942) -> (-7.3975, 64.7942)
  line L384 (-103.9199, 73.5933) -> (-108.25, 71.0933)
  line L385 (-108.25, 71.0933) -> (-108.25, 66.0933)
  line L386 (-108.25, 66.0933) -> (-103.9199, 63.5933)
  line L387 (-103.9199, 63.5933) -> (-99.5897, 66.0933)
  line L388 (-99.5897, 66.0933) -> (-99.5897, 71.0933)
  line L389 (-99.5897, 71.0933) -> (-103.9199, 73.5933)
  line L390 (-93.7596, 73.5933) -> (-98.0897, 71.0933)
  line L391 (-98.0897, 71.0933) -> (-98.0897, 66.0933)
  line L392 (-98.0897, 66.0933) -> (-93.7596, 63.5933)
  line L393 (-93.7596, 63.5933) -> (-89.4295, 66.0933)
  line L394 (-89.4295, 66.0933) -> (-89.4295, 71.0933)
  line L395 (-89.4295, 71.0933) -> (-93.7596, 73.5933)
  line L396 (-83.5994, 73.5933) -> (-87.9295, 71.0933)
  line L397 (-87.9295, 71.0933) -> (-87.9295, 66.0933)
  line L398 (-87.9295, 66.0933) -> (-83.5994, 63.5933)
  line L399 (-83.5994, 63.5933) -> (-79.2692, 66.0933)
  line L400 (-79.2692, 66.0933) -> (-79.2692, 71.0933)
  line L401 (-79.2692, 71.0933) -> (-83.5994, 73.5933)
  line L402 (-73.4391, 73.5933) -> (-77.7692, 71.0933)
  line L403 (-77.7692, 71.0933) -> (-77.7692, 66.0933)
  line L404 (-77.7692, 66.0933) -> (-73.4391, 63.5933)
  line L405 (-73.4391, 63.5933) -> (-69.109, 66.0933)
  line L406 (-69.109, 66.0933) -> (-69.109, 71.0933)
  line L407 (-69.109, 71.0933) -> (-73.4391, 73.5933)
  line L408 (-63.2789, 73.5933) -> (-67.609, 71.0933)
  line L409 (-67.609, 71.0933) -> (-67.609, 66.0933)
  line L410 (-67.609, 66.0933) -> (-63.2789, 63.5933)
  line L411 (-63.2789, 63.5933) -> (-58.9487, 66.0933)
  line L412 (-58.9487, 66.0933) -> (-58.9487, 71.0933)
  line L413 (-58.9487, 71.0933) -> (-63.2789, 73.5933)
  line L414 (-53.1186, 73.5933) -> (-57.4487, 71.0933)
  line L415 (-57.4487, 71.0933) -> (-57.4487, 66.0933)
  line L416 (-57.4487, 66.0933) -> (-53.1186, 63.5933)
  line L417 (-53.1186, 63.5933) -> (-48.7885, 66.0933)
  line L418 (-48.7885, 66.0933) -> (-48.7885, 71.0933)
  line L419 (-48.7885, 71.0933) -> (-53.1186, 73.5933)
  line L420 (-42.9584, 73.5933) -> (-47.2885, 71.0933)
  line L421 (-47.2885, 71.0933) -> (-47.2885, 66.0933)
  line L422 (-47.2885, 66.0933) -> (-42.9584, 63.5933)
  line L423 (-42.9584, 63.5933) -> (-38.6282, 66.0933)
  line L424 (-38.6282, 66.0933) -> (-38.6282, 71.0933)
  line L425 (-38.6282, 71.0933) -> (-42.9584, 73.5933)
  line L426 (-32.7981, 73.5933) -> (-37.1282, 71.0933)
  line L427 (-37.1282, 71.0933) -> (-37.1282, 66.0933)
  line L428 (-37.1282, 66.0933) -> (-32.7981, 63.5933)
  line L429 (-32.7981, 63.5933) -> (-28.468, 66.0933)
  line L430 (-28.468, 66.0933) -> (-28.468, 71.0933)
  line L431 (-28.468, 71.0933) -> (-32.7981, 73.5933)
  line L432 (-22.6378, 73.5933) -> (-26.968, 71.0933)
  line L433 (-26.968, 71.0933) -> (-26.968, 66.0933)
  line L434 (-26.968, 66.0933) -> (-22.6378, 63.5933)
  line L435 (-22.6378, 63.5933) -> (-18.3077, 66.0933)
  line L436 (-18.3077, 66.0933) -> (-18.3077, 71.0933)
  line L437 (-18.3077, 71.0933) -> (-22.6378, 73.5933)
  line L438 (-12.4776, 73.5933) -> (-16.8077, 71.0933)
  line L439 (-16.8077, 71.0933) -> (-16.8077, 66.0933)
  line L440 (-16.8077, 66.0933) -> (-12.4776, 63.5933)
  line L441 (-12.4776, 63.5933) -> (-8.1475, 66.0933)
  line L442 (-8.1475, 66.0933) -> (-8.1475, 71.0933)
  line L443 (-8.1475, 71.0933) -> (-12.4776, 73.5933)
  line L444 (-109, 82.3923) -> (-113.3301, 79.8923)
  line L445 (-113.3301, 79.8923) -> (-113.3301, 74.8923)
  line L446 (-113.3301, 74.8923) -> (-109, 72.3923)
  line L447 (-109, 72.3923) -> (-104.6699, 74.8923)
  line L448 (-104.6699, 74.8923) -> (-104.6699, 79.8923)
  line L449 (-104.6699, 79.8923) -> (-109, 82.3923)
  line L450 (-98.8397, 82.3923) -> (-103.1699, 79.8923)
  line L451 (-103.1699, 79.8923) -> (-103.1699, 74.8923)
  line L452 (-103.1699, 74.8923) -> (-98.8397, 72.3923)
  line L453 (-98.8397, 72.3923) -> (-94.5096, 74.8923)
  line L454 (-94.5096, 74.8923) -> (-94.5096, 79.8923)
  line L455 (-94.5096, 79.8923) -> (-98.8397, 82.3923)
  line L456 (-88.6795, 82.3923) -> (-93.0096, 79.8923)
  line L457 (-93.0096, 79.8923) -> (-93.0096, 74.8923)
  line L458 (-93.0096, 74.8923) -> (-88.6795, 72.3923)
  line L459 (-88.6795, 72.3923) -> (-84.3494, 74.8923)
  line L460 (-84.3494, 74.8923) -> (-84.3494, 79.8923)
  line L461 (-84.3494, 79.8923) -> (-88.6795, 82.3923)
  line L462 (-78.5192, 82.3923) -> (-82.8494, 79.8923)
  line L463 (-82.8494, 79.8923) -> (-82.8494, 74.8923)
  line L464 (-82.8494, 74.8923) -> (-78.5192, 72.3923)
  line L465 (-78.5192, 72.3923) -> (-74.1891, 74.8923)
  line L466 (-74.1891, 74.8923) -> (-74.1891, 79.8923)
  line L467 (-74.1891, 79.8923) -> (-78.5192, 82.3923)
  line L468 (-68.359, 82.3923) -> (-72.6891, 79.8923)
  line L469 (-72.6891, 79.8923) -> (-72.6891, 74.8923)
  line L470 (-72.6891, 74.8923) -> (-68.359, 72.3923)
  line L471 (-68.359, 72.3923) -> (-64.0289, 74.8923)
  line L472 (-64.0289, 74.8923) -> (-64.0289, 79.8923)
  line L473 (-64.0289, 79.8923) -> (-68.359, 82.3923)
  line L474 (-58.1987, 82.3923) -> (-62.5289, 79.8923)
  line L475 (-62.5289, 79.8923) -> (-62.5289, 74.8923)
  line L476 (-62.5289, 74.8923) -> (-58.1987, 72.3923)
  line L477 (-58.1987, 72.3923) -> (-53.8686, 74.8923)
  line L478 (-53.8686, 74.8923) -> (-53.8686, 79.8923)
  line L479 (-53.8686, 79.8923) -> (-58.1987, 82.3923)
  line L480 (-48.0385, 82.3923) -> (-52.3686, 79.8923)
  line L481 (-52.3686, 79.8923) -> (-52.3686, 74.8923)
  line L482 (-52.3686, 74.8923) -> (-48.0385, 72.3923)
  line L483 (-48.0385, 72.3923) -> (-43.7084, 74.8923)
  line L484 (-43.7084, 74.8923) -> (-43.7084, 79.8923)
  line L485 (-43.7084, 79.8923) -> (-48.0385, 82.3923)
  line L486 (-37.8782, 82.3923) -> (-42.2084, 79.8923)
  line L487 (-42.2084, 79.8923) -> (-42.2084, 74.8923)
  line L488 (-42.2084, 74.8923) -> (-37.8782, 72.3923)
  line L489 (-37.8782, 72.3923) -> (-33.5481, 74.8923)
  line L490 (-33.5481, 74.8923) -> (-33.5481, 79.8923)
  line L491 (-33.5481, 79.8923) -> (-37.8782, 82.3923)
  line L492 (-27.718, 82.3923) -> (-32.0481, 79.8923)
  line L493 (-32.0481, 79.8923) -> (-32.0481, 74.8923)
  line L494 (-32.0481, 74.8923) -> (-27.718, 72.3923)
  line L495 (-27.718, 72.3923) -> (-23.3878, 74.8923)
  line L496 (-23.3878, 74.8923) -> (-23.3878, 79.8923)
  line L497 (-23.3878, 79.8923) -> (-27.718, 82.3923)
  line L498 (-17.5577, 82.3923) -> (-21.8878, 79.8923)
  line L499 (-21.8878, 79.8923) -> (-21.8878, 74.8923)
  line L500 (-21.8878, 74.8923) -> (-17.5577, 72.3923)
  line L501 (-17.5577, 72.3923) -> (-13.2276, 74.8923)
  line L502 (-13.2276, 74.8923) -> (-13.2276, 79.8923)
  line L503 (-13.2276, 79.8923) -> (-17.5577, 82.3923)
  line L504 (-7.3975, 82.3923) -> (-11.7276, 79.8923)
  line L505 (-11.7276, 79.8923) -> (-11.7276, 74.8923)
  line L506 (-11.7276, 74.8923) -> (-7.3975, 72.3923)
  line L507 (-7.3975, 72.3923) -> (-3.0673, 74.8923)
  line L508 (-3.0673, 74.8923) -> (-3.0673, 79.8923)
  line L509 (-3.0673, 79.8923) -> (-7.3975, 82.3923)
  line L510 (-103.9199, 91.1913) -> (-108.25, 88.6913)
  line L511 (-108.25, 88.6913) -> (-108.25, 83.6913)
  line L512 (-108.25, 83.6913) -> (-103.9199, 81.1913)
  line L513 (-103.9199, 81.1913) -> (-99.5897, 83.6913)
  line L514 (-99.5897, 83.6913) -> (-99.5897, 88.6913)
  line L515 (-99.5897, 88.6913) -> (-103.9199, 91.1913)
  line L516 (-93.7596, 91.1913) -> (-98.0897, 88.6913)
  line L517 (-98.0897, 88.6913) -> (-98.0897, 83.6913)
  line L518 (-98.0897, 83.6913) -> (-93.7596, 81.1913)
  line L519 (-93.7596, 81.1913) -> (-89.4295, 83.6913)
  line L520 (-89.4295, 83.6913) -> (-89.4295, 88.6913)
  line L521 (-89.4295, 88.6913) -> (-93.7596, 91.1913)
  line L522 (-83.5994, 91.1913) -> (-87.9295, 88.6913)
  line L523 (-87.9295, 88.6913) -> (-87.9295, 83.6913)
  line L524 (-87.9295, 83.6913) -> (-83.5994, 81.1913)
  line L525 (-83.5994, 81.1913) -> (-79.2692, 83.6913)
  line L526 (-79.2692, 83.6913) -> (-79.2692, 88.6913)
  line L527 (-79.2692, 88.6913) -> (-83.5994, 91.1913)
  line L528 (-73.4391, 91.1913) -> (-77.7692, 88.6913)
  line L529 (-77.7692, 88.6913) -> (-77.7692, 83.6913)
  line L530 (-77.7692, 83.6913) -> (-73.4391, 81.1913)
  line L531 (-73.4391, 81.1913) -> (-69.109, 83.6913)
  line L532 (-69.109, 83.6913) -> (-69.109, 88.6913)
  line L533 (-69.109, 88.6913) -> (-73.4391, 91.1913)
  line L534 (-63.2789, 91.1913) -> (-67.609, 88.6913)
  line L535 (-67.609, 88.6913) -> (-67.609, 83.6913)
  line L536 (-67.609, 83.6913) -> (-63.2789, 81.1913)
  line L537 (-63.2789, 81.1913) -> (-58.9487, 83.6913)
  line L538 (-58.9487, 83.6913) -> (-58.9487, 88.6913)
  line L539 (-58.9487, 88.6913) -> (-63.2789, 91.1913)
  line L540 (-53.1186, 91.1913) -> (-57.4487, 88.6913)
  line L541 (-57.4487, 88.6913) -> (-57.4487, 83.6913)
  line L542 (-57.4487, 83.6913) -> (-53.1186, 81.1913)
  line L543 (-53.1186, 81.1913) -> (-48.7885, 83.6913)
  line L544 (-48.7885, 83.6913) -> (-48.7885, 88.6913)
  line L545 (-48.7885, 88.6913) -> (-53.1186, 91.1913)
  line L546 (-42.9584, 91.1913) -> (-47.2885, 88.6913)
  line L547 (-47.2885, 88.6913) -> (-47.2885, 83.6913)
  line L548 (-47.2885, 83.6913) -> (-42.9584, 81.1913)
  line L549 (-42.9584, 81.1913) -> (-38.6282, 83.6913)
  line L550 (-38.6282, 83.6913) -> (-38.6282, 88.6913)
  line L551 (-38.6282, 88.6913) -> (-42.9584, 91.1913)
  line L552 (-32.7981, 91.1913) -> (-37.1282, 88.6913)
  line L553 (-37.1282, 88.6913) -> (-37.1282, 83.6913)
  line L554 (-37.1282, 83.6913) -> (-32.7981, 81.1913)
  line L555 (-32.7981, 81.1913) -> (-28.468, 83.6913)
  line L556 (-28.468, 83.6913) -> (-28.468, 88.6913)
  line L557 (-28.468, 88.6913) -> (-32.7981, 91.1913)
  line L558 (-22.6378, 91.1913) -> (-26.968, 88.6913)
  line L559 (-26.968, 88.6913) -> (-26.968, 83.6913)
  line L560 (-26.968, 83.6913) -> (-22.6378, 81.1913)
  line L561 (-22.6378, 81.1913) -> (-18.3077, 83.6913)
  line L562 (-18.3077, 83.6913) -> (-18.3077, 88.6913)
  line L563 (-18.3077, 88.6913) -> (-22.6378, 91.1913)
  line L564 (-12.4776, 91.1913) -> (-16.8077, 88.6913)
  line L565 (-16.8077, 88.6913) -> (-16.8077, 83.6913)
  line L566 (-16.8077, 83.6913) -> (-12.4776, 81.1913)
  line L567 (-12.4776, 81.1913) -> (-8.1475, 83.6913)
  line L568 (-8.1475, 83.6913) -> (-8.1475, 88.6913)
  line L569 (-8.1475, 88.6913) -> (-12.4776, 91.1913)
  line L570 (-109, 99.9904) -> (-113.3301, 97.4904)
  line L571 (-113.3301, 97.4904) -> (-113.3301, 92.4904)
  line L572 (-113.3301, 92.4904) -> (-109, 89.9904)
  line L573 (-109, 89.9904) -> (-104.6699, 92.4904)
  line L574 (-104.6699, 92.4904) -> (-104.6699, 97.4904)
  line L575 (-104.6699, 97.4904) -> (-109, 99.9904)
  line L576 (-98.8397, 99.9904) -> (-103.1699, 97.4904)
  line L577 (-103.1699, 97.4904) -> (-103.1699, 92.4904)
  line L578 (-103.1699, 92.4904) -> (-98.8397, 89.9904)
  line L579 (-98.8397, 89.9904) -> (-94.5096, 92.4904)
  line L580 (-94.5096, 92.4904) -> (-94.5096, 97.4904)
  line L581 (-94.5096, 97.4904) -> (-98.8397, 99.9904)
  line L582 (-88.6795, 99.9904) -> (-93.0096, 97.4904)
  line L583 (-93.0096, 97.4904) -> (-93.0096, 92.4904)
  line L584 (-93.0096, 92.4904) -> (-88.6795, 89.9904)
  line L585 (-88.6795, 89.9904) -> (-84.3494, 92.4904)
  line L586 (-84.3494, 92.4904) -> (-84.3494, 97.4904)
  line L587 (-84.3494, 97.4904) -> (-88.6795, 99.9904)
  line L588 (-78.5192, 99.9904) -> (-82.8494, 97.4904)
  line L589 (-82.8494, 97.4904) -> (-82.8494, 92.4904)
  line L590 (-82.8494, 92.4904) -> (-78.5192, 89.9904)
  line L591 (-78.5192, 89.9904) -> (-74.1891, 92.4904)
  line L592 (-74.1891, 92.4904) -> (-74.1891, 97.4904)
  line L593 (-74.1891, 97.4904) -> (-78.5192, 99.9904)
  line L594 (-68.359, 99.9904) -> (-72.6891, 97.4904)
  line L595 (-72.6891, 97.4904) -> (-72.6891, 92.4904)
  line L596 (-72.6891, 92.4904) -> (-68.359, 89.9904)
  line L597 (-68.359, 89.9904) -> (-64.0289, 92.4904)
  line L598 (-64.0289, 92.4904) -> (-64.0289, 97.4904)
  line L599 (-64.0289, 97.4904) -> (-68.359, 99.9904)
  line L600 (-58.1987, 99.9904) -> (-62.5289, 97.4904)
  line L601 (-62.5289, 97.4904) -> (-62.5289, 92.4904)
  line L602 (-62.5289, 92.4904) -> (-58.1987, 89.9904)
  line L603 (-58.1987, 89.9904) -> (-53.8686, 92.4904)
  line L604 (-53.8686, 92.4904) -> (-53.8686, 97.4904)
  line L605 (-53.8686, 97.4904) -> (-58.1987, 99.9904)
  line L606 (-48.0385, 99.9904) -> (-52.3686, 97.4904)
  line L607 (-52.3686, 97.4904) -> (-52.3686, 92.4904)
  line L608 (-52.3686, 92.4904) -> (-48.0385, 89.9904)
  line L609 (-48.0385, 89.9904) -> (-43.7084, 92.4904)
  line L610 (-43.7084, 92.4904) -> (-43.7084, 97.4904)
  line L611 (-43.7084, 97.4904) -> (-48.0385, 99.9904)
  line L612 (-37.8782, 99.9904) -> (-42.2084, 97.4904)
  line L613 (-42.2084, 97.4904) -> (-42.2084, 92.4904)
  line L614 (-42.2084, 92.4904) -> (-37.8782, 89.9904)
  line L615 (-37.8782, 89.9904) -> (-33.5481, 92.4904)
  line L616 (-33.5481, 92.4904) -> (-33.5481, 97.4904)
  line L617 (-33.5481, 97.4904) -> (-37.8782, 99.9904)
  line L618 (-27.718, 99.9904) -> (-32.0481, 97.4904)
  line L619 (-32.0481, 97.4904) -> (-32.0481, 92.4904)
  line L620 (-32.0481, 92.4904) -> (-27.718, 89.9904)
  line L621 (-27.718, 89.9904) -> (-23.3878, 92.4904)
  line L622 (-23.3878, 92.4904) -> (-23.3878, 97.4904)
  line L623 (-23.3878, 97.4904) -> (-27.718, 99.9904)
  line L624 (-17.5577, 99.9904) -> (-21.8878, 97.4904)
  line L625 (-21.8878, 97.4904) -> (-21.8878, 92.4904)
  line L626 (-21.8878, 92.4904) -> (-17.5577, 89.9904)
  line L627 (-17.5577, 89.9904) -> (-13.2276, 92.4904)
  line L628 (-13.2276, 92.4904) -> (-13.2276, 97.4904)
  line L629 (-13.2276, 97.4904) -> (-17.5577, 99.9904)
  line L630 (-7.3975, 99.9904) -> (-11.7276, 97.4904)
  line L631 (-11.7276, 97.4904) -> (-11.7276, 92.4904)
  line L632 (-11.7276, 92.4904) -> (-7.3975, 89.9904)
  line L633 (-7.3975, 89.9904) -> (-3.0673, 92.4904)
  line L634 (-3.0673, 92.4904) -> (-3.0673, 97.4904)
  line L635 (-3.0673, 97.4904) -> (-7.3975, 99.9904)
  line L636 (-103.9199, 108.7894) -> (-108.25, 106.2894)
  line L637 (-108.25, 106.2894) -> (-108.25, 101.2894)
  line L638 (-108.25, 101.2894) -> (-103.9199, 98.7894)
  line L639 (-103.9199, 98.7894) -> (-99.5897, 101.2894)
  line L640 (-99.5897, 101.2894) -> (-99.5897, 106.2894)
  line L641 (-99.5897, 106.2894) -> (-103.9199, 108.7894)
  line L642 (-93.7596, 108.7894) -> (-98.0897, 106.2894)
  line L643 (-98.0897, 106.2894) -> (-98.0897, 101.2894)
  line L644 (-98.0897, 101.2894) -> (-93.7596, 98.7894)
  line L645 (-93.7596, 98.7894) -> (-89.4295, 101.2894)
  line L646 (-89.4295, 101.2894) -> (-89.4295, 106.2894)
  line L647 (-89.4295, 106.2894) -> (-93.7596, 108.7894)
  line L648 (-83.5994, 108.7894) -> (-87.9295, 106.2894)
  line L649 (-87.9295, 106.2894) -> (-87.9295, 101.2894)
  line L650 (-87.9295, 101.2894) -> (-83.5994, 98.7894)
  line L651 (-83.5994, 98.7894) -> (-79.2692, 101.2894)
  line L652 (-79.2692, 101.2894) -> (-79.2692, 106.2894)
  line L653 (-79.2692, 106.2894) -> (-83.5994, 108.7894)
  line L654 (-73.4391, 108.7894) -> (-77.7692, 106.2894)
  line L655 (-77.7692, 106.2894) -> (-77.7692, 101.2894)
  line L656 (-77.7692, 101.2894) -> (-73.4391, 98.7894)
  line L657 (-73.4391, 98.7894) -> (-69.109, 101.2894)
  line L658 (-69.109, 101.2894) -> (-69.109, 106.2894)